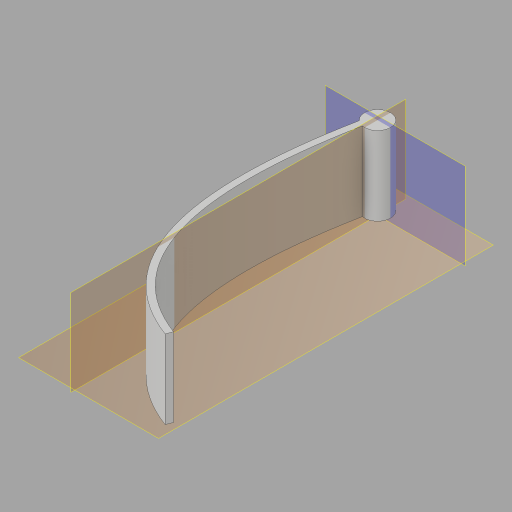
# Autodesk Inventor part: Strap for Pflanzenwagen
Saved by Autodesk Inventor 2023.2 (Build 272271000, 271)
## iProperties
Created: 2023-02-01
Part Number: Strap for Pflanzenwagen
Material: Generisch
Document SubType Name: Modeling
Designer: Raoul Messerli
Density: 1 g/cm^3
Appearance: Vorgabe
Author: Raoul Messerli
Autodesk Inventor part; units mm, degrees
sketch "Skizze4" plane through (0, 0, 0) normal (0, 0, 1) x (1, 0, 0)
  circle A0 centre (0, 0) radius 6.5981
  constraints: 1 centre point, 1 coincident
extrude "Extrusion4" add sketch "Skizze4" along normal blind 40
sketch "Skizze5" plane through (0, 0, 0) normal (0, 0, 1) x (1, 0, 0)
  circle A0 centre (0, 0) radius 6.5981 projected
  line L0 (0, 0) -> (-25.1787, -120.4123) construction
  line L1 (-25.1787, -120.4123) -> (41.3959, -145.3028) construction
  spline S0 degree 2 poles (0, 0) (-25.1787, -120.4123) (41.3959, -145.3028) knots 1 1 1 2 2 2
  line L2 (41.3959, -145.3028) -> (40.2355, -148.4065)
  spline S1 degree 5 poles (-3.2433, 0.6782) (-5.0976, -8.1898) (-6.7208, -17.1063) (-8.072, -26.0707) (-9.9466, -42.5339) (-10.43, -59.0918) (-10.3114, -66.594) (-9.343, -80.3525) (-6.645, -93.8689) (-5.0006, -99.939) (-0.949, -111.1448) (5.0395, -121.4318) (8.327, -126.0068) (15.8459, -134.436) (24.934, -141.1438) (29.8297, -144.0248) (34.9512, -146.4307) (40.2355, -148.4065) knots 0 0 0 0 0 0 0.266037 0.266037 0.266037 0.486055 0.486055 0.486055 0.67009 0.67009 0.67009 0.834347 0.834347 0.834347 1 1 1 1 1 1
  point P0 (-1.2997, -6.4688)
  point P1 (-4.3779, -4.9364)
  constraints: 2 end point, 1 perpendicular, 6 other
extrude "Extrusion5" add sketch "Skizze5" along normal blind 40 contours A0 S0 L2 S1
